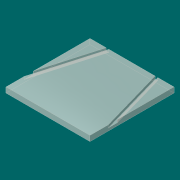
# Autodesk Inventor part: topBottom
Saved by Autodesk Inventor 2016 (Build 200138000, 138)
## iProperties
Created: 2015-10-13
Part Number: topBottom
Material: PC/ABS Plastic
Document SubType Name: Modeling
Designer: Sawaiz
Density: 0.357273 g/cm^3
Appearance: Clear
Author: Sawaiz
Autodesk Inventor part; units mm, degrees
ref_plane "YZ Plane" through (0, 0, 0) normal (1, 0, 0) x (0, 1, 0)
ref_plane "XZ Plane" through (0, 0, 0) normal (0, 1, 0) x (-1, 0, 0)
ref_plane "XY Plane" through (0, 0, 0) normal (0, 0, 1) x (1, 0, 0)
sketch "Sketch1" plane through (0, 0, 0) normal (0, 0, 1) x (1, 0, 0)
  line L0 (-50, -50) -> (50, -50)
  line L1 (50, -50) -> (50, 50)
  line L2 (50, 50) -> (-50, 50)
  line L3 (-50, 50) -> (-50, -50)
  line L4 (-50, -50) -> (50, 50) construction
  line L5 (50, -50) -> (-50, 50) construction
  point P0 (0, 0)
  dimension "d0" = 100
  dimension "d1" = 100
  constraints: 12 end point, 2 midpoint, 2 parallel, 1 horizontal, 1 perpendicular
  measures "d0" distance of L2.end L1.end
  measures "d1" distance of L1.end L0.end
extrude "Extrusion1" add sketch "Sketch1" along normal blind 6.35
sketch "Sketch3" plane through (0, 0, 6.35) normal (0, 0, 1) x (1, 0, 0)
  line L0 (-50, -50) -> (50, -50) projected
  line L1 (50, -50) -> (50, 50) projected
  line L2 (50, 50) -> (-50, 50) projected
  line L3 (-50, 50) -> (-50, -50) projected
  line L4 (-50, -50) -> (50, -50) projected
  line L5 (28.376, -53.1209) -> (-50, -30.6469)
  line L6 (28.376, -50) -> (-50, -27.526)
  line L7 (-50, 27.526) -> (28.376, 50)
  line L8 (50, -50) -> (50, 50) projected
  line L9 (28.376, 53.1209) -> (-50, 30.6469)
  line L10 (50, 50) -> (-50, 50) projected
  line L11 (-50, 50) -> (-50, -50) projected
  line L12 (-50, -27.526) -> (-50, 27.526)
  line L13 (28.376, 53.1209) -> (28.376, -53.1209)
  point P0 (0, 0)
  point P1 (-50, 0)
  dimension "d10" = 3
  dimension "d11" = 3
  dimension "d15" = 16
  dimension "d16" = 21.624
  constraints: 12 end point, 9 point on line, 2 midpoint, 2 parallel, 1 collinear, 1 vertical
  measures "d10" distance between parallel lines of L7 L9
  measures "d11" distance between parallel lines of L5 L6
  measures "d15" angle of L0 L5
  measures "d16" distance between parallel lines of L1 L13
extrude "Extrusion2" cut sketch "Sketch3" against normal blind 3.175 contours L13 L5 L0 | L0 L5 L3 L6 | L7 L3 L9 L2 | L2 L9 L13
equation "\"d0\" = depth"
equation "\"d1\" = width"
equation "\"d2\" = acrylicThickness"
equation "\"d10\" = mirrorThickness"
equation "\"d11\" = mirrorThickness"
equation "\"d15\" = mirrorAngle"
equation "\"d16\" = centerThickness + aerogelThickness + fresnelThickness"
equation "\"d7\" = 0.5 * acrylicThickness"
equation "\"acrylicThickness\" = 6.35"
equation "\"width\" = 100"
equation "\"depth\" = 100"
equation "\"mirrorAngle\" = 16deg"
equation "\"mirrorThickness\" = 3"
equation "\"aerogelThickness\" = 20"
equation "\"detectorWidth\" = 52"
equation "\"detectorHeight\" = 52"
equation "\"fresnelThickness\" = 0.1"
equation "\"focalLength\" = 76.2"
equation "\"ior\" = 1.49"
equation "\"centerThickness\" = 1.524"
equation "\"fresnelAngle\" = 90deg"
equation "\"fresnelEffectiveDiameter\" = 76.2"
body "Solid1"
